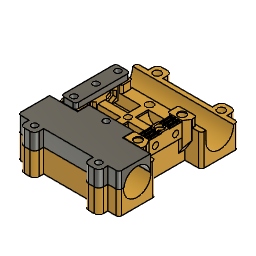
X_Carriage_Brassv7 (Autodesk Fusion 360 design; units mm, degrees)
Autodesk Fusion 360 part; units mm, degrees
note: some values were not read from the file. Set by a fixed rule: which face or edge a step refers to.
sketch "スケッチ1" plane through (0, 0, 0) normal (0, 0, 1) x (1, 0, 0)
  line L0 (-27.5, 32.5) -> (27.5, 32.5)
  line L1 (27.5, 32.5) -> (27.5, 12.5)
  line L2 (27.5, 12.5) -> (18.5, 12.5)
  line L3 (18.5, 12.5) -> (18.5, -12.5)
  line L4 (18.5, -12.5) -> (27.5, -12.5)
  line L5 (27.5, -12.5) -> (27.5, -32.5)
  line L6 (27.5, -32.5) -> (-27.5, -32.5)
  line L7 (-27.5, -32.5) -> (-27.5, -12.5)
  line L8 (-27.5, -12.5) -> (-18.5, -12.5)
  line L9 (-18.5, -12.5) -> (-18.5, 12.5)
  line L10 (-18.5, 12.5) -> (-27.5, 12.5)
  line L11 (-27.5, 12.5) -> (-27.5, 32.5)
  circle A0 centre (0, 0) radius 1.75
  dimension "d1" = 55
  dimension "d2" = 65
  dimension "d3" = 20
  dimension "d4" = 20
  dimension "d5" = 9
  dimension "d6" = 27.5
  dimension "d7" = 32.5
  dimension "d8" = 9
  dimension "d9" = 3.5
  constraint perpendicular L0 L1
  constraint perpendicular L1 L2
  constraint perpendicular L2 L3
  constraint perpendicular L1 L4
  constraint perpendicular L4 L5
  constraint perpendicular L5 L6
  constraint perpendicular L4 L7
  constraint perpendicular L7 L8
  constraint perpendicular L8 L9
  constraint perpendicular L9 L10
  constraint perpendicular L0 L11
  constraint collinear L2 L10
  constraint collinear L4 L8
  constraint collinear L1 L5
  constraint collinear L7 L11
  constraint horizontal L0
  constraint coincident A0.centre origin
  measures "d1" horizontal distance of L5.end L6.end
  measures "d2" distance of L0 L6
  measures "d3" vertical distance of L0.end L1.end
  measures "d4" vertical distance of L4.end L5.end
  measures "d5" horizontal distance of L1.end L2.end
  measures "d6" distance of A0.centre L5
  measures "d7" distance of A0.centre L0
  measures "d8" horizontal distance of L9.end L10.end
  measures "d9" diameter of A0
extrude "押し出し1" add sketch "スケッチ1" along normal blind 17.3 makes body 1
sketch "スケッチ2" plane through (27.5, 0, 0) normal (1, 0, 0) x (0, 1, 0)
  line L0 (12.5, 0) -> (32.5, 0)
  line L1 (32.5, 0) -> (32.5, 17.3)
  line L2 (32.5, 17.3) -> (12.5, 17.3)
  line L3 (12.5, 17.3) -> (12.5, 0)
  line L4 (22.5, 0) -> (22.5, 17.3) construction
  line L5 (12.5, 12.6228) -> (32.5, 12.6228) construction
  circle A0 centre (22.5, 12) radius 7.495
  line L6 (32.5, 12.6228) -> (29.7996, 17.3)
  line L7 (32.5, 12.6228) -> (38.6199, 12.6228) construction
  line L8 (12.5, 12.6228) -> (15.2004, 17.3)
  line L9 (12.5, 17.3) -> (-12.5, 17.3)
  line L10 (0, 0) -> (0, 17.3) construction
  circle A1 centre (-22.5, 12) radius 7.495
  line L11 (-12.5, 12.6228) -> (-15.2004, 17.3)
  line L12 (-32.5, 12.6228) -> (-29.7996, 17.3)
  line L13 (-32.5, 17.3) -> (-12.5, 17.3)
  line L14 (-32.5, 0) -> (-32.5, 17.3)
  line L15 (-12.5, 17.3) -> (-12.5, 0)
  line L16 (12.5, 12.6228) -> (32.5, 12.6228)
  line L17 (-32.5, 12.6228) -> (-12.5, 12.6228)
  point P0 (0, 17.3)
  dimension "d12" = 12.6228
  dimension "d13" = 14.99
  dimension "d14" = 120
  dimension "d15" = 60
  dimension "d135" = 12
  constraint midpoint L0 L4.start
  constraint midpoint L2 L4.end
  constraint coincident L3 L5.start
  constraint coincident L1 L5.end
  constraint perpendicular L1 L5
  constraint coincident L2 L6.end
  constraint horizontal L7
  constraint coincident L2 L8.end
  constraint coincident L4 A0.centre
  constraint coincident L10.start origin
  constraint coincident P0 L10.end
  constraint symmetric L5.start L10 L11.start
  constraint symmetric L5.end L10 L12.start
  constraint symmetric A0 L10 A1
  constraint symmetric L6.end L10 L12.end
  constraint symmetric L8.end L10 L11.end
  constraint symmetric L0.start L10 L15.end
  constraint symmetric L0.end L10 L14.start
  constraint symmetric L1.end L10 L13.start
  constraint symmetric L2.end L10 L9.end
  measures "d12" distance of L0 L5
  measures "d13" diameter of A0
  measures "d14" angle of L6 L7
  measures "d15" angle of L7 L8
  measures "d135" distance of L4.start A0.centre
extrude "押し出し2" cut sketch "スケッチ2" against normal blind 55 contours L2 L3 L8 | L2 A0 L8 L16 | L1 L2 L6 | L2 A0 L6 L16 | A0 L16 | L2 A0 L16 | A1 L17 | A1 L13 L17 | A1 L11 L13 L17 | A1 L12 L13 L17 | L11 L13 L15 | L12 L13 L14 bodies 1
extrude "押し出し3" cut sketch "スケッチ2" against normal blind 9 contours L2 L3 L8 | L11 L13 L15 bodies 1
extrude "押し出し4" cut sketch "スケッチ2" against normal blind 9 from surface at -46 contours L2 L3 L8 | L11 L13 L15 bodies 1
sketch "スケッチ3" plane through (0, 0, 17.3) normal (0, 0, 1) x (-1, 0, 0)
  line L0 (18.5, -12.5) -> (18.5, 12.5)
  line L1 (-18.5, 12.5) -> (-18.5, -12.5)
  circle A0 centre (0, 0) radius 1.75
  line L2 (-12.5, -15.0033) -> (-12.5, -9)
  line L3 (-2, -9) -> (-22.5, -9)
  line L4 (-22.5, -9) -> (-22.5, -15.0033)
  line L5 (-22.5, -15.0033) -> (-12.5, -15.0033)
  line L6 (-2, -9) -> (-2, -2)
  line L7 (-2, -2) -> (-18.5, -2)
  line L8 (-18.5, -12.5) -> (18.5, -12.5)
  line L9 (18.5, 12.5) -> (-18.5, 12.5)
  dimension "d23" = 10
  dimension "d24" = 12.5
  dimension "d26" = 7
  dimension "d27" = 2
  dimension "d28" = 16.5
  constraint perpendicular L2 L3
  constraint vertical L6
  constraint coincident L1 L7.end
  constraint perpendicular L1 L7
  constraint coincident L2.end L3
  measures "d23" horizontal distance of L2.start L4.end
  measures "d24" horizontal distance of A0.centre L2.start
  measures "d26" vertical distance of L6.end L3.start
  measures "d27" distance of A0.centre L7
  measures "d28" horizontal distance of L6.end L7.end
extrude "押し出し5" cut sketch "スケッチ3" against normal blind 5.9 contours L1 L3 L6 L7 bodies 1
fillet "フィレット3" radius 5 1 edges at (2, 5.5, 11.4) on bodies 1
mirror "ミラー1" about plane through (0, 0, 0) normal (0, 1, 0) of "押し出し5", "フィレット3"
mirror "ミラー2" about plane through (0, 0, 0) normal (1, 0, 0) of "押し出し5", "フィレット3", "ミラー1"
extrude "押し出し6" add sketch "スケッチ3" against normal blind 12.3 separate body contours L1 L2 L3 L8 | L1 L2 L3 L4 L5 L8 makes body 2
chamfer "面取り2" distance 4 distance2 6.4 1 edges at (22.5, 12.0016, 5) measured on face at (17.8333, 13.0022, 5) on bodies 2
extrude "押し出し7" add sketch "スケッチ3" along normal blind 4.1 contours L1 L2 L3 L8 | L1 L2 L3 L4 L5 L8 bodies 2
chamfer "面取り3" distance 2 distance2 3.5 1 edges at (22.5, 9, 16.4) measured on face at (15.8333, 9, 12.6) on bodies 2
sketch "スケッチ4" plane through (0, 0, 21.4) normal (0, 0, 1) x (-1, 0, 0)
  line L0 (-20.5, -9) -> (-22.5, -12.5)
  line L1 (-22.5, -12.5) -> (-22.5, -15.0033)
  line L2 (-22.5, -15.0033) -> (-12.5, -15.0033)
  line L3 (-12.5, -15.0033) -> (-12.5, -9)
  line L4 (-12.5, -9) -> (-20.5, -9)
  line L5 (-17.5, -9) -> (-17.5, -15.0033) construction
  line L6 (-22.5, -12.5) -> (-12.5, -12.5) construction
  circle A0 centre (-17.5, -12.5) radius 1.75
  circle A1 centre (-17.5, -12.5) radius 2.35
  circle A2 centre (-17.5, -12.5) radius 2.5
  dimension "d47" = 3.5
  dimension "d48" = 5
  dimension "d50" = 5
  dimension "d51" = 4.7
  dimension "d53" = 3.5
  constraint coincident L4 L5.start
  constraint coincident L2 L5.end
  constraint coincident L1 L0.end
  constraint coincident L3 L6.end
  constraint perpendicular L4 L5
  constraint perpendicular L3 L6
  constraint midpoint L6 A0.centre
  constraint concentric A0 A1
  constraint concentric A1 A2
  measures "d47" distance of L3.end L6.end
  measures "d48" distance of L1 L5
  measures "d50" diameter of A2
  measures "d51" diameter of A1
  measures "d53" diameter of A0
fillet "フィレット1" radius 1 4 edges at (12.5, 9, 13.2) (12.5, 15.0033, 13.2) (22.5, 15.0033, 16.4) (22.5, 12.5, 16.4) on bodies 2
extrude "押し出し19" cut sketch "スケッチ2" against normal blind 20 contours A0 L16 | L2 A0 L16 bodies 2
mirror "ミラー3" about plane through (0, 0, 0) normal (0, 1, 0) of bodies 2 makes body 3
sketch "スケッチ5" plane through (0, 9, 0) normal (0, -1, 0) x (1, 0, 0)
  line L0 (13.5, 21.4) -> (13.5, 5)
  line L1 (13.5, 5) -> (18.5, 5)
  line L2 (18.5, 5) -> (20.5, 8.2)
  line L3 (20.5, 8.2) -> (20.5, 21.4)
  line L4 (20.5, 21.4) -> (13.5, 21.4)
  line L5 (13.5, 13.4) -> (20.5, 13.4)
  line L6 (14.5, 13.4) -> (14.5, 21.4)
  line L7 (20.5, 20.95) -> (14.5, 20.95)
  line L8 (17.5, 20.95) -> (17.5, 20.2) construction
  arc A0 (17.0011, 20.5118) -> (17.9989, 20.5118) centre (17.5, 20.755) ccw
  arc A1 (16.9, 20.95) -> (17.0011, 20.5118) centre (17.9, 20.95) ccw
  arc A2 (17.9989, 20.5118) -> (18.1, 20.95) centre (17.1, 20.95) ccw
  arc A3 (15.9989, 20.5118) -> (16.1, 20.95) centre (15.1, 20.95) ccw
  arc A4 (15.0011, 20.5118) -> (15.9989, 20.5118) centre (15.5, 20.755) ccw
  arc A5 (14.9, 20.95) -> (15.0011, 20.5118) centre (15.9, 20.95) ccw
  arc A6 (19.9989, 20.5118) -> (20.1, 20.95) centre (19.1, 20.95) ccw
  arc A7 (19.0011, 20.5118) -> (19.9989, 20.5118) centre (19.5, 20.755) ccw
  arc A8 (18.9, 20.95) -> (19.0011, 20.5118) centre (19.9, 20.95) ccw
  dimension "d62" = 8
  dimension "d63" = 6
  dimension "d64" = 0.45
  dimension "d65" = 0.75
  dimension "d70" = 0.555
  dimension "d71" = 1
  dimension "d72" = 1
  dimension "d75" = 2
  dimension "d76" = 0
  constraint coincident L0 L5.start
  constraint coincident L3 L5.end
  constraint perpendicular L0 L5
  constraint coincident L5 L6.start
  constraint coincident L4 L6.end
  constraint perpendicular L5 L6
  constraint coincident L3 L7.start
  constraint coincident L6 L7.end
  constraint perpendicular L6 L7
  constraint midpoint L7 L8.start
  constraint vertical L8
  constraint coincident L8 A0.centre
  constraint coincident L7 A1.centre
  constraint coincident L7 A2.centre
  constraint coincident L7 A1.start
  constraint coincident L7 A2.end
  constraint coincident L8.end A0
  constraint tangent A0 A1
  constraint coincident A0.start A1.end
  constraint coincident A0.end A2.start
  constraint tangent A0 A2
  measures "d62" distance of L4 L5
  measures "d63" distance of L3 L6
  measures "d64" distance of L4 L7
  measures "d65" distance of L8.start L8.end
  measures "d70" radius of A0
  measures "d71" radius of A1
  measures "d72" radius of A2
extrude "押し出し11" add sketch "スケッチ5" along normal up to surface (18 mm away) contours L3 L5 L6 L7 A0 A1 A2 A3 A4 A5 A6 A7 A8 bodies 2 3
fillet "フィレット2" radius 0.15 6 edges at (14.9, 0, 20.95) (16.1, 0, 20.95) (16.9, 0, 20.95) (18.1, 0, 20.95) (18.9, 0, 20.95) (20.1, 0, 20.95) on bodies 2
sketch "スケッチ6" plane through (0, 0, 13.4) normal (0, 0, -1) x (1, 0, 0)
  line L0 (20.5, 9) -> (14.5, 9)
  line L1 (14.5, 9) -> (14.5, -9)
  line L2 (14.5, -9) -> (20.5, -9)
  line L3 (20.5, -9) -> (20.5, 9)
  line L4 (14.5, 0) -> (20.5, 0) construction
  line L5 (14.5, 2) -> (20.5, 2)
  line L6 (14.5, -2) -> (20.5, -2)
  dimension "d87" = 2
  dimension "d88" = 2
  constraint midpoint L1 L4.start
  constraint midpoint L3 L4.end
  constraint coincident L1 L5.start
  constraint coincident L3 L5.end
  constraint perpendicular L3 L5
  constraint coincident L1 L6.start
  constraint coincident L3 L6.end
  constraint perpendicular L3 L6
  measures "d87" distance of L4 L5
  measures "d88" distance of L4 L6
extrude "押し出し15" add sketch "スケッチ6" against normal blind 8 contours L1 L3 L5 L6 bodies 2
sketch "スケッチ7" plane through (0, 0, 21.4) normal (0, 0, 1) x (-1, 0, 0)
  line L0 (-14.5, -2) -> (-14.5, 2)
  line L1 (-14.5, 2) -> (-20.5, 2)
  line L2 (-20.5, 2) -> (-20.5, -2)
  line L3 (-20.5, -2) -> (-14.5, -2)
  line L4 (-14.5, 0) -> (-20.5, 0) construction
  circle A0 centre (-17.5, 0) radius 1.75
  circle A1 centre (-17.5, 0) radius 2.05
  circle A2 centre (-17.5, 0) radius 2.15
  dimension "d91" = 3.5
  dimension "d92" = 4.1
  dimension "d93" = 4.3
  constraint midpoint L0 L4.start
  constraint midpoint L2 L4.end
  constraint midpoint L4 A0.centre
  constraint concentric A0 A1
  constraint concentric A1 A2
  measures "d91" diameter of A0
  measures "d92" diameter of A1
  measures "d93" diameter of A2
sketch "スケッチ8" plane through (20.5, 0, 0) normal (1, 0, 0) x (0, 1, 0)
  line L0 (-9, 13.4) -> (9, 13.4)
  line L1 (9, 13.4) -> (9, 20.95)
  line L2 (9, 20.95) -> (2, 20.95)
  line L3 (2, 20.95) -> (2, 21.4)
  line L4 (2, 21.4) -> (-2, 21.4)
  line L5 (-2, 21.4) -> (-2, 20.95)
  line L6 (-2, 20.95) -> (-9, 20.95)
  line L7 (-9, 20.95) -> (-9, 13.4)
  line L8 (9, 16.9) -> (-9, 16.9) construction
  line L9 (5.5, 13.4) -> (5.5, 20.95) construction
  circle A0 centre (5.5, 16.9) radius 1.65
  dimension "d104" = 3.5
  dimension "d105" = 3.5
  dimension "d106" = 3.3
  constraint coincident L7 L8.end
  constraint coincident L0 L9.start
  constraint coincident L2 L9.end
  constraint perpendicular L2 L9
  constraint coincident L8 A0.centre
  constraint coincident L9 A0.centre
  measures "d104" distance of L1 L9
  measures "d105" distance of L0 L8
  measures "d106" diameter of A0
extrude "押し出し20" cut sketch "スケッチ8" against normal blind 10 contours A0 bodies 2
extrude "押し出し21" cut sketch "スケッチ8" against normal blind 0.5 contours A0 bodies 2
mirror "ミラー6" about plane through (0, 0, 0) normal (0, 1, 0) of "押し出し20", "押し出し21"
mirror "ミラー5" about plane through (0, 0, 0) normal (1, 0, 0) of bodies 2 makes body 4
combine "結合1" operation add target body 1 tool bodies 2 4
sketch "スケッチ9" plane through (0, 0, 21.4) normal (0, 0, 1) x (-1, 0, 0)
  arc A0 (-22.3682, -12.2694) -> (-22.5, -12.7656) centre (-21.5, -12.7656) ccw
  line L0 (-22.5, -12.7656) -> (-22.5, -14.0033)
  arc A1 (-22.5, -14.0033) -> (-21.5, -15.0033) centre (-21.5, -14.0033) ccw
  line L1 (-21.5, -15.0033) -> (-13.5, -15.0033)
  arc A2 (-13.5, -15.0033) -> (-12.5, -14.0033) centre (-13.5, -14.0033) ccw
  line L2 (-12.5, -14.0033) -> (-12.5, -10)
  arc A3 (-12.5, -10) -> (-13.5, -9) centre (-13.5, -10) ccw
  line L3 (-13.5, -9) -> (-20.5, -9)
  line L4 (-20.5, -9) -> (-22.3682, -12.2694)
  line L5 (-12.5, -12.0016) -> (-22.5, -12.0016) construction
  line L6 (-17.5, -15.0033) -> (-17.5, -9) construction
  circle A4 centre (-17.5, -12.0016) radius 1.75
  circle A5 centre (-17.5, -12.0016) radius 2.05
  circle A6 centre (-17.5, -12.0016) radius 2.15
  dimension "d113" = 5
  dimension "d115" = 4.3
  dimension "d116" = 4.1
  dimension "d117" = 3.5
  constraint coincident L2 L5.start
  constraint coincident L0 L5.end
  constraint coincident L1 L6.start
  constraint perpendicular L1 L6
  constraint perpendicular L2 L5
  constraint midpoint L5 A4.centre
  constraint concentric A4 A5
  constraint concentric A5 A6
  constraint coincident L3 L6.end
  constraint midpoint L2 L5.start
  measures "d113" distance of L2 L6
  measures "d115" diameter of A6
  measures "d116" diameter of A5
  measures "d117" diameter of A4
extrude "押し出し22" cut sketch "スケッチ9" against normal blind 14 contours A4 bodies 1
extrude "押し出し23" cut sketch "スケッチ9" against normal blind 5 contours A5 bodies 1
extrude "押し出し24" cut sketch "スケッチ9" against normal blind 0.5 contours A6 bodies 1
mirror "ミラー7" about plane through (0, 0, 0) normal (0, 1, 0) of "押し出し22", "押し出し23", "押し出し24"
mirror "ミラー8" about plane through (0, 0, 0) normal (1, 0, 0) of "押し出し22", "押し出し23", "押し出し24", "ミラー7"
extrude "押し出し25" cut sketch "スケッチ7" against normal blind 7.6 contours A0 bodies 1
extrude "押し出し26" cut sketch "スケッチ7" against normal blind 6 contours L3 A1 | L1 L3 A1 | L1 A1 bodies 1
extrude "押し出し27" cut sketch "スケッチ7" against normal blind 1.5 contours L3 A1 A2 | L1 L3 A1 A2 | L1 A1 A2 | L1 L3 A1 A2 bodies 1
mirror "ミラー9" about plane through (0, 0, 0) normal (1, 0, 0) of "押し出し25", "押し出し26", "押し出し27"
sketch "スケッチ10" plane through (0, 0, 0) normal (0, 0, -1) x (1, 0, 0)
  circle A0 centre (0, 0) radius 1.75
  line L0 (27.5, 12.5) -> (27.5, 32.5)
  line L1 (27.5, 32.5) -> (-27.5, 32.5)
  line L2 (-27.5, 32.5) -> (-27.5, 12.5)
  line L3 (-27.5, 12.5) -> (-18.5, 12.5)
  line L4 (-18.5, 12.5) -> (-18.5, -12.5)
  line L5 (-18.5, -12.5) -> (-27.5, -12.5)
  line L6 (-27.5, -12.5) -> (-27.5, -32.5)
  line L7 (-27.5, -32.5) -> (27.5, -32.5)
  line L8 (27.5, -32.5) -> (27.5, -12.5)
  line L9 (27.5, -12.5) -> (18.5, -12.5)
  line L10 (18.5, -12.5) -> (18.5, 12.5)
  line L11 (18.5, 12.5) -> (27.5, 12.5)
  circle A1 centre (12, 12) radius 2.05
  circle A2 centre (-12, 12) radius 2.05
  circle A3 centre (-12, -12) radius 2.05
  circle A4 centre (12, -12) radius 2.05
  dimension "d139" = 4.1
  dimension "d140" = 12
  dimension "d141" = 12
  dimension "d143" = 360
  measures "d139" diameter of A1
  measures "d140" horizontal distance of A0.centre A1.centre
  measures "d141" vertical distance of A0.centre A1.centre
extrude "押し出し28" cut sketch "スケッチ10" against normal blind 10 contours A1 | A2 | A3 | A4 bodies 1
sketch "Sketch11" plane through (14.5, 0, 0) normal (-1, 0, 0) x (0, -1, 0)
  line L0 (-2, 13.4) -> (-2, 17.3)
  line L1 (-2, 17.3) -> (2, 17.3)
  line L2 (2, 17.3) -> (2, 13.4)
  line L3 (2, 13.4) -> (9, 13.4)
  line L4 (9, 13.4) -> (9, 20.95)
  line L5 (9, 20.95) -> (2, 20.95)
  line L6 (2, 20.95) -> (2, 21.4)
  line L7 (2, 21.4) -> (-2, 21.4)
  line L8 (-2, 21.4) -> (-2, 20.95)
  line L9 (-2, 20.95) -> (-9, 20.95)
  line L10 (-9, 20.95) -> (-9, 13.4)
  line L11 (-9, 13.4) -> (-2, 13.4)
  circle A0 centre (-5.5, 16.9) radius 1.65
  circle A1 centre (5.5, 16.9) radius 1.65
  line L12 (8.3, 18.5166) -> (5.5, 20.1332)
  line L13 (5.5, 20.1332) -> (2.7, 18.5166)
  line L14 (2.7, 18.5166) -> (2.7, 15.2834)
  line L15 (2.7, 15.2834) -> (5.5, 13.6668)
  line L16 (5.5, 13.6668) -> (8.3, 15.2834)
  line L17 (8.3, 15.2834) -> (8.3, 18.5166)
  line L18 (0, 0) -> (0, 31.0723) construction
  line L19 (0, 2.5) -> (0, 20)
  line L20 (0, 0) -> (0, 31.0723) construction
  line L21 (-2.7, 18.5166) -> (-2.7, 15.2834)
  line L22 (-2.7, 15.2834) -> (-5.5, 13.6668)
  line L23 (-5.5, 13.6668) -> (-8.3, 15.2834)
  line L24 (-8.3, 15.2834) -> (-8.3, 18.5166)
  line L25 (-5.5, 20.1332) -> (-2.7, 18.5166)
  line L26 (-8.3, 18.5166) -> (-5.5, 20.1332)
  point P0 (5.5, 16.9)
  dimension "d147" = 2.8
  constraint coincident P0 A1.centre
  constraint vertical L14
  constraint coincident L18.start L20.start
  constraint vertical L18
  constraint symmetric L12.start L19 L24.end
  constraint symmetric L12.end L19 L25.start
  constraint symmetric L13.end L19 L21.start
  constraint symmetric L14.end L19 L21.end
  constraint symmetric L15.end L19 L22.end
  constraint symmetric L16.end L19 L23.end
  constraint symmetric L18.start L19 L20.start
  constraint symmetric L18.end L19 L20.end
  measures "d147" distance of P0 L17
extrude "Extrude29" cut sketch "Sketch11" against normal blind 2 contours L12 L13 L14 L15 L16 L17 | L21 L22 L23 L24 L25 L26 bodies 1
mirror "Mirror10" about plane through (0, 0, 0) normal (1, 0, 0) of "Extrude29"
sketch "Sketch12" plane through (0, 0, 12.6228) normal (0, 0, 1) x (-1, 0, 0)
  line L0 (-27.5, 32.5) -> (-27.5, 29.9691)
  line L1 (-27.5, 29.9691) -> (27.5, 29.9691)
  line L2 (27.5, 29.9691) -> (27.5, 32.5)
  line L3 (27.5, 32.5) -> (-27.5, 32.5)
  circle A0 centre (-17.5, -12.0016) radius 1.75
  circle A1 centre (17.5, -12.0016) radius 1.75
  line L4 (-17.5, -12.0016) -> (-17.5, 32.5) construction
  line L5 (17.5, -12.0016) -> (17.5, 32.5)
  line L6 (27.5, -32.5) -> (-27.5, -32.5)
  line L7 (-17.5, -12.0016) -> (-17.5, -32.5) construction
  line L8 (17.5, -12.0016) -> (17.5, -32.5) construction
  circle A2 centre (-17.5, 33.4691) radius 2.05
  line L9 (0, 0) -> (0, 39.6041) construction
  line L10 (-13.5, 29.9691) -> (-21.5, 29.9691)
  line L11 (-21.5, 29.9691) -> (-21.5, 37.4691)
  line L12 (-21.5, 37.4691) -> (-13.5, 37.4691)
  line L13 (-13.5, 37.4691) -> (-13.5, 29.9691)
  line L14 (13.5, 29.9691) -> (21.5, 29.9691)
  line L15 (21.5, 29.9691) -> (21.5, 37.4691)
  line L16 (13.5, 37.4691) -> (13.5, 29.9691)
  line L17 (21.5, 37.4691) -> (13.5, 37.4691)
  circle A3 centre (17.5, 33.4691) radius 2.05
  dimension "d151" = 4.1
  dimension "d152" = 3.5
  dimension "d153" = 4
  dimension "d154" = 4
  dimension "d155" = 4
  constraint coincident A0.centre L4.start
  constraint coincident L3 L4.end
  constraint perpendicular L3 L4
  constraint coincident A1.centre L5.start
  constraint coincident L3 L5.end
  constraint perpendicular L3 L5
  constraint coincident L6 L7.end
  constraint perpendicular L6 L7
  constraint coincident L6 L8.end
  constraint perpendicular L6 L8
  constraint coincident L4 A2.centre
  constraint coincident L9.start origin
  constraint perpendicular L1 L9
  constraint horizontal L10
  constraint vertical L11
  constraint horizontal L12
  constraint vertical L13
  constraint coincident L1 L10.start
  constraint symmetric A2 L9 A3
  constraint symmetric L9 L10.start L14.start
  constraint symmetric L9 L10.end L14.end
  constraint symmetric L9 L11.end L15.end
  constraint symmetric L9 L12.end L16.start
  measures "d151" diameter of A2
  measures "d152" distance of L1 A2.centre
  measures "d153" distance of A2.centre L11
  measures "d154" distance of A2.centre L13
  measures "d155" distance of A2.centre L12
extrude "Extrude30" add sketch "Sketch12" against normal up to surface (12.6228 mm away) contours L3 A2 L11 L12 L13 | L3 L15 L16 L17 A3 bodies 1
extrude "Extrude31" cut sketch "Sketch12" against normal up to surface (12.6228 mm away) contours L3 A2 | L3 L5 A3 | L3 L5 A3 picked at (-17.7101, 31.915) bodies 1
sketch "Sketch13" plane through (0, 0, 0) normal (0, 0, -1) x (1, 0, 0)
  circle A0 centre (17.5, 33.4691) radius 2.05
  circle A1 centre (-17.5, 33.4691) radius 2.05
  line L0 (13.5, 32.5) -> (-13.5, 32.5)
  line L1 (-13.5, 32.5) -> (-13.5, 37.4691)
  line L2 (-13.5, 37.4691) -> (-21.5, 37.4691)
  line L3 (-21.5, 37.4691) -> (-21.5, 32.5)
  line L4 (-21.5, 32.5) -> (-27.5, 32.5)
  line L5 (-27.5, 32.5) -> (-27.5, 12.5)
  line L6 (-27.5, 12.5) -> (-18.5, 12.5)
  line L7 (-18.5, 12.5) -> (-18.5, -12.5)
  line L8 (-18.5, -12.5) -> (-27.5, -12.5)
  line L9 (-27.5, -12.5) -> (-27.5, -32.5)
  line L10 (-27.5, -32.5) -> (27.5, -32.5)
  line L11 (27.5, -32.5) -> (27.5, -12.5)
  line L12 (27.5, -12.5) -> (18.5, -12.5)
  line L13 (18.5, -12.5) -> (18.5, 12.5)
  line L14 (18.5, 12.5) -> (27.5, 12.5)
  line L15 (27.5, 12.5) -> (27.5, 32.5)
  line L16 (27.5, 32.5) -> (21.5, 32.5)
  line L17 (21.5, 32.5) -> (21.5, 37.4691)
  line L18 (21.5, 37.4691) -> (13.5, 37.4691)
  line L19 (13.5, 37.4691) -> (13.5, 32.5)
  circle A2 centre (12, -12) radius 2.05
  circle A3 centre (-12, -12) radius 2.05
  circle A4 centre (12, 12) radius 2.05
  circle A5 centre (-12, 12) radius 2.05
  circle A6 centre (0, 0) radius 1.75
extrude "Extrude32" add sketch "Sketch13" against normal up to surface (4.6228 mm away) contours A0 | A1 bodies 1
mirror "Mirror11" about plane through (0, 0, 0) normal (0, 1, 0) of "Extrude30", "Extrude31", "Extrude32"
fillet "Fillet6" radius 2.5 8 edges at (-21.5, -37.4691, 6.3114) (21.5, -37.4691, 6.3114) (13.5, -37.4691, 6.3114) (-13.5, -37.4691, 6.3114) (-21.5, 37.4691, 6.3114) (-13.5, 37.4691, 6.3114) (13.5, 37.4691, 6.3114) (21.5, 37.4691, 6.3114) on bodies 1
extrude "Extrude4" add 1 faces at (-25.5, -31.6564, 12.6228) along direction (0, 0, 1) up to surface (8.7772 mm away) separate body on bodies 1 makes body 5 in component "Component"
extrude "Extrude33" add 1 faces at (-25.8333, -13.8447, 12.6228) along direction (0, 0, 1) up to surface (4.6772 mm away) on bodies 1 bodies 1
extrude "Extrude34" add 1 faces at (-25.8333, 13.8447, 12.6228) along direction (0, 0, 1) up to surface (4.6772 mm away) on bodies 1 bodies 1
sketch "Sketch14" plane through (0, 0, 17.3) normal (0, 0, 1) x (-1, 0, 0)
  circle A0 centre (0, 0) radius 1.75
  line L0 (14.5, -2) -> (14.5, 2)
  line L1 (14.5, 2) -> (2, 2)
  line L2 (2, 2) -> (2, 9)
  line L3 (2, 9) -> (13.5, 9)
  arc A1 (12.5, 10) -> (13.5, 9) centre (13.5, 10) ccw
  line L4 (12.5, 10) -> (12.5, 14.0033)
  arc A2 (13.5, 15.0033) -> (12.5, 14.0033) centre (13.5, 14.0033) ccw
  line L5 (13.5, 15.0033) -> (21.5, 15.0033)
  arc A3 (22.5, 14.0033) -> (21.5, 15.0033) centre (21.5, 14.0033) ccw
  line L6 (22.5, 14.0033) -> (22.5, 12.7656)
  arc A4 (22.4641, 12.5) -> (22.5, 12.7656) centre (21.5, 12.7656) ccw
  line L7 (22.4641, 12.5) -> (27.5, 12.5)
  line L8 (27.5, 12.5) -> (27.5, 15.0309)
  line L9 (27.5, 15.0309) -> (-27.5, 15.0309)
  line L10 (-27.5, 15.0309) -> (-27.5, 12.5)
  line L11 (-27.5, 12.5) -> (-22.4641, 12.5)
  arc A5 (-22.5, 12.7656) -> (-22.4641, 12.5) centre (-21.5, 12.7656) ccw
  line L12 (-22.5, 12.7656) -> (-22.5, 14.0033)
  arc A6 (-21.5, 15.0033) -> (-22.5, 14.0033) centre (-21.5, 14.0033) ccw
  line L13 (-21.5, 15.0033) -> (-13.5, 15.0033)
  arc A7 (-12.5, 14.0033) -> (-13.5, 15.0033) centre (-13.5, 14.0033) ccw
  line L14 (-12.5, 14.0033) -> (-12.5, 10)
  arc A8 (-13.5, 9) -> (-12.5, 10) centre (-13.5, 10) ccw
  line L15 (-13.5, 9) -> (-2, 9)
  line L16 (-2, 9) -> (-2, 2)
  line L17 (-2, 2) -> (-14.5, 2)
  line L18 (-14.5, 2) -> (-14.5, -2)
  line L19 (-14.5, -2) -> (-2, -2)
  line L20 (-2, -2) -> (-2, -9)
  line L21 (-2, -9) -> (-13.5, -9)
  arc A9 (-12.5, -10) -> (-13.5, -9) centre (-13.5, -10) ccw
  line L22 (-12.5, -10) -> (-12.5, -14.0033)
  arc A10 (-13.5, -15.0033) -> (-12.5, -14.0033) centre (-13.5, -14.0033) ccw
  line L23 (-13.5, -15.0033) -> (-21.5, -15.0033)
  arc A11 (-22.5, -14.0033) -> (-21.5, -15.0033) centre (-21.5, -14.0033) ccw
  line L24 (-22.5, -14.0033) -> (-22.5, -12.7656)
  arc A12 (-22.4641, -12.5) -> (-22.5, -12.7656) centre (-21.5, -12.7656) ccw
  line L25 (-22.4641, -12.5) -> (-27.5, -12.5)
  line L26 (-27.5, -12.5) -> (-27.5, -15.0309)
  line L27 (-27.5, -15.0309) -> (27.5, -15.0309)
  line L28 (27.5, -15.0309) -> (27.5, -12.5)
  line L29 (27.5, -12.5) -> (22.4641, -12.5)
  arc A13 (22.5, -12.7656) -> (22.4641, -12.5) centre (21.5, -12.7656) ccw
  line L30 (22.5, -12.7656) -> (22.5, -14.0033)
  arc A14 (21.5, -15.0033) -> (22.5, -14.0033) centre (21.5, -14.0033) ccw
  line L31 (21.5, -15.0033) -> (13.5, -15.0033)
  arc A15 (12.5, -14.0033) -> (13.5, -15.0033) centre (13.5, -14.0033) ccw
  line L32 (12.5, -14.0033) -> (12.5, -10)
  arc A16 (13.5, -9) -> (12.5, -10) centre (13.5, -10) ccw
  line L33 (13.5, -9) -> (2, -9)
  line L34 (2, -9) -> (2, -2)
  line L35 (2, -2) -> (14.5, -2)
  circle A17 centre (0, 11.8) radius 2.05
  circle A18 centre (0, -11.8) radius 2.05
  line L36 (-26.2107, 0) -> (26.7893, 0) construction
  line L37 (0, -15.0309) -> (0, 15.0309) construction
  dimension "d179" = 4.1
  dimension "d180" = 4.1
  dimension "d181" = 2.8
  constraint horizontal L36
  constraint coincident A0.centre L36
  constraint symmetric A17.centre A18.centre L36
  constraint midpoint L27 L37.start
  constraint midpoint L9 L37.end
  constraint coincident A17.centre L37
  measures "d179" diameter of A17
  measures "d180" diameter of A18
  measures "d181" distance of L15 A17.centre
extrude "Extrude35" cut sketch "Sketch14" against normal blind 8 contours A17 | A18 bodies 1
sketch "Sketch4" plane through (0, 0, 17.3) normal (0, 0, 1) x (-1, 0, 0) in component "Component"
  circle A0 centre (0, 11.8) radius 2.05
  circle A1 centre (0, -11.8) radius 2.05
  circle A2 centre (0, 0) radius 1.75
  line L0 (14.5, -2) -> (14.5, 2)
  line L1 (14.5, 2) -> (2, 2)
  line L2 (2, 2) -> (2, 9)
  line L3 (2, 9) -> (13.5, 9)
  arc A3 (12.5, 10) -> (13.5, 9) centre (13.5, 10) ccw
  line L4 (12.5, 10) -> (12.5, 14.0033)
  arc A4 (13.5, 15.0033) -> (12.5, 14.0033) centre (13.5, 14.0033) ccw
  line L5 (13.5, 15.0033) -> (21.5, 15.0033)
  arc A5 (22.5, 14.0033) -> (21.5, 15.0033) centre (21.5, 14.0033) ccw
  line L6 (22.5, 14.0033) -> (22.5, 12.7656)
  arc A6 (22.4641, 12.5) -> (22.5, 12.7656) centre (21.5, 12.7656) ccw
  line L7 (22.4641, 12.5) -> (27.5, 12.5)
  line L8 (27.5, 12.5) -> (27.5, 15.0309)
  line L9 (27.5, 15.0309) -> (-27.5, 15.0309)
  line L10 (-27.5, 15.0309) -> (-27.5, 12.5)
  line L11 (-27.5, 12.5) -> (-22.4641, 12.5)
  arc A7 (-22.5, 12.7656) -> (-22.4641, 12.5) centre (-21.5, 12.7656) ccw
  line L12 (-22.5, 12.7656) -> (-22.5, 14.0033)
  arc A8 (-21.5, 15.0033) -> (-22.5, 14.0033) centre (-21.5, 14.0033) ccw
  line L13 (-21.5, 15.0033) -> (-13.5, 15.0033)
  arc A9 (-12.5, 14.0033) -> (-13.5, 15.0033) centre (-13.5, 14.0033) ccw
  line L14 (-12.5, 14.0033) -> (-12.5, 10)
  arc A10 (-13.5, 9) -> (-12.5, 10) centre (-13.5, 10) ccw
  line L15 (-13.5, 9) -> (-2, 9)
  line L16 (-2, 9) -> (-2, 2)
  line L17 (-2, 2) -> (-14.5, 2)
  line L18 (-14.5, 2) -> (-14.5, -2)
  line L19 (-14.5, -2) -> (-2, -2)
  line L20 (-2, -2) -> (-2, -9)
  line L21 (-2, -9) -> (-13.5, -9)
  arc A11 (-12.5, -10) -> (-13.5, -9) centre (-13.5, -10) ccw
  line L22 (-12.5, -10) -> (-12.5, -14.0033)
  arc A12 (-13.5, -15.0033) -> (-12.5, -14.0033) centre (-13.5, -14.0033) ccw
  line L23 (-13.5, -15.0033) -> (-21.5, -15.0033)
  arc A13 (-22.5, -14.0033) -> (-21.5, -15.0033) centre (-21.5, -14.0033) ccw
  line L24 (-22.5, -14.0033) -> (-22.5, -12.7656)
  arc A14 (-22.4641, -12.5) -> (-22.5, -12.7656) centre (-21.5, -12.7656) ccw
  line L25 (-22.4641, -12.5) -> (-27.5, -12.5)
  line L26 (-27.5, -12.5) -> (-27.5, -15.0309)
  line L27 (-27.5, -15.0309) -> (27.5, -15.0309)
  line L28 (27.5, -15.0309) -> (27.5, -12.5)
  line L29 (27.5, -12.5) -> (22.4641, -12.5)
  arc A15 (22.5, -12.7656) -> (22.4641, -12.5) centre (21.5, -12.7656) ccw
  line L30 (22.5, -12.7656) -> (22.5, -14.0033)
  arc A16 (21.5, -15.0033) -> (22.5, -14.0033) centre (21.5, -14.0033) ccw
  line L31 (21.5, -15.0033) -> (13.5, -15.0033)
  arc A17 (12.5, -14.0033) -> (13.5, -15.0033) centre (13.5, -14.0033) ccw
  line L32 (12.5, -14.0033) -> (12.5, -10)
  arc A18 (13.5, -9) -> (12.5, -10) centre (13.5, -10) ccw
  line L33 (13.5, -9) -> (2, -9)
  line L34 (2, -9) -> (2, -2)
  line L35 (2, -2) -> (14.5, -2)
  line L36 (2, 9) -> (13.5, 9)
  line L37 (-13.5, 9) -> (-2, 9)
  line L38 (-27.5, 15.0309) -> (27.5, 15.0309)
  line L39 (12.5, 14.0033) -> (12.5, 10)
  line L40 (-12.5, 14.0033) -> (-12.5, 10)
  line L41 (12.5, 9) -> (-12.5, 9)
  line L42 (-12.5, 9) -> (-12.5, 15.0309)
  line L43 (-12.5, 15.0309) -> (12.5, 15.0309)
  line L44 (12.5, 15.0309) -> (12.5, 9)
  circle A19 centre (0, 11.8) radius 1.65
  dimension "d187" = 3.3
  constraint horizontal L41
  constraint vertical L42
  constraint horizontal L43
  constraint vertical L44
  constraint coincident L9 L42.end
  constraint coincident L3 L41.start
  constraint collinear L14 L42
  constraint collinear L39 L44
  constraint concentric A0 A19
  measures "d187" diameter of A19
extrude "Extrude5" add sketch "Sketch4" along normal up to surface (4.1 mm away) separate body contours A0 | L3 L4 L9 L14 L15 L36 L37 L38 L39 L40 L41 L42 L43 L44 makes body 6 in component "Component"
move_face "OffsetFaces4" offset -0.2 6 faces at (-12.5, -9.6667, 18.6667) (-12.5, -11.3344, 20.0333) (-12.5, -14.6884, 18.6667) (12.5, -14.3458, 18.6667) (12.5, -12.6689, 18.6667) (12.5, -9.3333, 18.6667) on bodies 6 in component "Component"
move_face "OffsetFaces5" offset 0.4 2 faces at (-15.799, -32.3249, 18.4743) (15.471, -33.7619, 18.4743) on bodies 5 in component "Component"
sketch "Sketch5" plane through (27.5, 0, 0) normal (1, 0, 0) x (0, 1, 0) in component "Component"
  line L0 (-29.9691, 21.4) -> (-32.5, 21.4)
  line L1 (-32.5, 21.4) -> (-32.5, 12.6228)
  line L2 (-32.5, 12.6228) -> (-29.9691, 12.6228)
  line L3 (-29.9691, 12.6228) -> (-29.9691, 21.4)
  arc A0 (-29.9691, 12.6228) -> (-15.0309, 12.6228) centre (-22.5, 12) ccw
  circle A1 centre (-22.5, 12) radius 7.195
  line L4 (-29.9691, 12.6228) -> (-15.25, 12.6228)
  line L5 (-15.25, 12.6228) -> (-15.25, 21.4)
  line L6 (-15.25, 21.4) -> (-29.9691, 21.4)
  line L7 (-29.9691, 21.4) -> (-29.9691, 12.6228)
  dimension "d189" = 0.3
  constraint concentric A0 A1
  constraint horizontal L4
  constraint vertical L5
  constraint horizontal L6
  constraint vertical L7
  constraint coincident L2.end L3.start
  constraint coincident L0.start L3.end
  measures "d189" distance of A0 A1
extrude "Extrude6" add sketch "Sketch5" against normal up to surface (55 mm away) contours L3 A1 L4 L5 L6 L7 bodies 6 5 in component "Component"
extrude "Extrude7" add 1 faces at (-4.1, -15.0309, 18.6667) along direction (0, -1, 0) up to surface (0.2191 mm away) on bodies 6 bodies 6 5 in component "Component"
fillet "Fillet7" radius 1.5 8 edges at (27.5, -32.5, 6.3114) (-27.5, -32.5, 6.3114) (-27.5, -12.5, 8.65) (-27.5, 12.5, 8.65) (-27.5, 32.5, 6.3114) (27.5, 32.5, 6.3114) (27.5, 12.5, 8.65) (27.5, -12.5, 8.65) on bodies 1
fillet "Fillet1" radius 1.5 2 edges at (27.5, -32.5, 17.0114) (-27.5, -32.5, 17.0114) on bodies 6 in component "Component"
sketch "Sketch1" plane through (0, 0, 21.4) normal (0, 0, 1) x (-1, 0, 0) in component "clamp"
  circle A0 centre (-17.5, -12.0016) radius 2.15
  arc A1 (-22.3682, -12.2694) -> (-22.5, -12.7656) centre (-21.5, -12.7656) ccw
  line L0 (-22.5, -12.7656) -> (-22.5, -14.0033)
  arc A2 (-22.5, -14.0033) -> (-21.5, -15.0033) centre (-21.5, -14.0033) ccw
  line L1 (-21.5, -15.0033) -> (-13.5, -15.0033)
  arc A3 (-13.5, -15.0033) -> (-12.5, -14.0033) centre (-13.5, -14.0033) ccw
  line L2 (-12.5, -14.0033) -> (-12.5, -10)
  arc A4 (-12.5, -10) -> (-13.5, -9) centre (-13.5, -10) ccw
  line L3 (-13.5, -9) -> (-20.5, -9)
  line L4 (-20.5, -9) -> (-22.3682, -12.2694)
  line L5 (21.5, -14.7533) -> (13.5, -14.7533)
  line L6 (13.5, -14.7533) -> (13.5, 15)
  line L7 (13.5, 15) -> (21.5, 15)
  line L8 (21.5, 15) -> (21.5, -14.7533)
  line L9 (21.5, -15.0033) -> (13.5, -15.0033)
  line L10 (12.3, 15.25) -> (27.5, 15.25)
  circle A5 centre (17.5, 12.0016) radius 2.15
  circle A6 centre (17.5, -12.0016) radius 2.15
  circle A7 centre (17.5, 0) radius 2.05
  circle A8 centre (17.5, -12.0016) radius 1.65
  circle A9 centre (17.5, 0) radius 1.65
  circle A10 centre (17.5, 12.0016) radius 1.65
  line L11 (17.5, -14.7533) -> (17.5, 15) construction
  dimension "d196" = 0.25
  dimension "d197" = 0.25
  dimension "d198" = 3.3
  dimension "d199" = 3.3
  dimension "d200" = 3.3
  dimension "d203" = 8
  constraint horizontal L5
  constraint vertical L6
  constraint horizontal L7
  constraint vertical L8
  constraint concentric A6 A8
  constraint concentric A7 A9
  constraint concentric A5 A10
  constraint midpoint L5 L11.start
  constraint midpoint L7 L11.end
  constraint coincident A7.centre L11
  measures "d196" distance of L5 L9
  measures "d197" distance of L7 L10
  measures "d198" diameter of A8
  measures "d199" diameter of A9
  measures "d200" diameter of A10
  measures "d203" distance of L6 L8
extrude "Extrude1" add sketch "Sketch1" along normal blind 3 separate body contours L5 L6 L7 L8 | A5 | A6 | A7 makes body 7 in component "clamp"
fillet "Fillet1'" radius 1.5 4 edges at (-21.5, -15, 22.9) (-13.5, -15, 22.9) (-21.5, 14.7533, 22.9) (-13.5, 14.7533, 22.9) on bodies 7 in component "clamp"
sketch "Sketch15" plane through (0, 0, 0) normal (0, 0, -1) x (1, 0, 0)
  circle A0 centre (12, -12) radius 2.05
  circle A1 centre (-12, -12) radius 2.05
  circle A2 centre (12, 12) radius 2.05
  circle A3 centre (-12, 12) radius 2.05
  circle A4 centre (0, 0) radius 1.75
  arc A5 (26, 12.5) -> (27.5, 14) centre (26, 14) ccw
  line L0 (27.5, 14) -> (27.5, 31)
  arc A6 (27.5, 31) -> (26, 32.5) centre (26, 31) ccw
  line L1 (26, 32.5) -> (21.5, 32.5)
  line L2 (21.5, 32.5) -> (21.5, 34.9691)
  arc A7 (21.5, 34.9691) -> (19, 37.4691) centre (19, 34.9691) ccw
  line L3 (19, 37.4691) -> (16, 37.4691)
  arc A8 (16, 37.4691) -> (13.5, 34.9691) centre (16, 34.9691) ccw
  line L4 (13.5, 34.9691) -> (13.5, 32.5)
  line L5 (13.5, 32.5) -> (-13.5, 32.5)
  line L6 (-13.5, 32.5) -> (-13.5, 34.9691)
  arc A9 (-13.5, 34.9691) -> (-16, 37.4691) centre (-16, 34.9691) ccw
  line L7 (-16, 37.4691) -> (-19, 37.4691)
  arc A10 (-19, 37.4691) -> (-21.5, 34.9691) centre (-19, 34.9691) ccw
  line L8 (-21.5, 34.9691) -> (-21.5, 32.5)
  line L9 (-21.5, 32.5) -> (-26, 32.5)
  arc A11 (-26, 32.5) -> (-27.5, 31) centre (-26, 31) ccw
  line L10 (-27.5, 31) -> (-27.5, 14)
  arc A12 (-27.5, 14) -> (-26, 12.5) centre (-26, 14) ccw
  line L11 (-26, 12.5) -> (-18.5, 12.5)
  line L12 (-18.5, 12.5) -> (-18.5, -12.5)
  line L13 (-18.5, -12.5) -> (-26, -12.5)
  arc A13 (-26, -12.5) -> (-27.5, -14) centre (-26, -14) ccw
  line L14 (-27.5, -14) -> (-27.5, -31)
  arc A14 (-27.5, -31) -> (-26, -32.5) centre (-26, -31) ccw
  line L15 (-26, -32.5) -> (-21.5, -32.5)
  line L16 (-21.5, -32.5) -> (-21.5, -34.9691)
  arc A15 (-21.5, -34.9691) -> (-19, -37.4691) centre (-19, -34.9691) ccw
  line L17 (-19, -37.4691) -> (-16, -37.4691)
  arc A16 (-16, -37.4691) -> (-13.5, -34.9691) centre (-16, -34.9691) ccw
  line L18 (-13.5, -34.9691) -> (-13.5, -32.5)
  line L19 (-13.5, -32.5) -> (13.5, -32.5)
  line L20 (13.5, -32.5) -> (13.5, -34.9691)
  arc A17 (13.5, -34.9691) -> (16, -37.4691) centre (16, -34.9691) ccw
  line L21 (16, -37.4691) -> (19, -37.4691)
  arc A18 (19, -37.4691) -> (21.5, -34.9691) centre (19, -34.9691) ccw
  line L22 (21.5, -34.9691) -> (21.5, -32.5)
  line L23 (21.5, -32.5) -> (26, -32.5)
  arc A19 (26, -32.5) -> (27.5, -31) centre (26, -31) ccw
  line L24 (27.5, -31) -> (27.5, -14)
  arc A20 (27.5, -14) -> (26, -12.5) centre (26, -14) ccw
  line L25 (26, -12.5) -> (18.5, -12.5)
  line L26 (18.5, -12.5) -> (18.5, 12.5)
  line L27 (18.5, 12.5) -> (26, 12.5)
  circle A21 centre (12, -12) radius 2.05
  circle A22 centre (-12, -12) radius 2.05
  dimension "d205" = 4.1
  dimension "d206" = 4.1
  constraint concentric A0 A21
  constraint concentric A1 A22
  measures "d205" diameter of A21
  measures "d206" diameter of A22
extrude "Extrude36" cut sketch "Sketch15" against normal blind 6 contours A0 A21 | A1 A22 bodies 1
move_face "OffsetFaces6" [suppressed] in component "Component"
component "Component" placed x (1, 0, 0) y (0, 1, 0) z (0, 0, 1) at (0, 0, 0)
component "clamp" placed x (1, 0, 0) y (0, 1, 0) z (0, 0, 1) at (0, 0, 0)
equation "d6 = d1 / 2"
equation "d7 = d2 / 2"
equation "d8 = d5"
equation "d147 = ( 5.6 / 2 ) * 1 mm"
